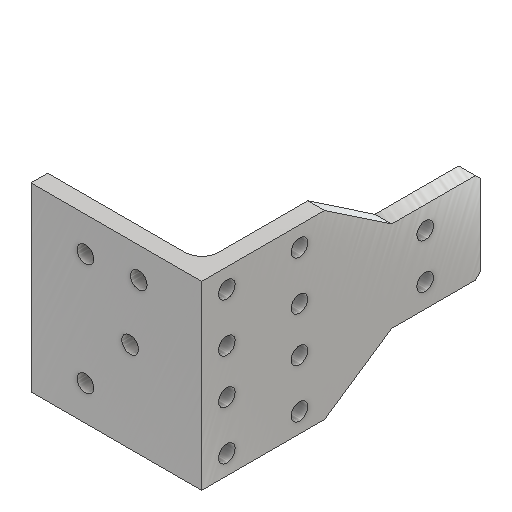
# Autodesk Inventor part: CNCM_X_Axiss_Carriage_Belt_and_Cable_Chain_Mount
Saved by Autodesk Inventor 2026.1 (Build 301233000, 233)
## iProperties
Created: 2016-03-27
Part Number: CNCM_X_Axiss_Carriage_Belt_and_Cable_Chain_Mount
Material: Ogólny
Document SubType Name: Modeling
Designer: Andrzej
Density: 1 g/cm^3
Appearance: Obrobione - aluminium
Mass: 6.52184 g
Surface Area: 50.6141 cm^2
Volume: 6.52184 cm^3
Author: Andrzej
Autodesk Inventor part; units mm, degrees
ref_plane "YZ Plane" through (0, 0, 0) normal (1, 0, 0) x (0, 1, 0)
ref_plane "XZ Plane" through (0, 0, 0) normal (0, 1, 0) x (-1, 0, 0)
ref_plane "XY Plane" through (0, 0, 0) normal (0, 0, 1) x (1, 0, 0)
sketch "Szkic1" plane through (0, 0, 0) normal (0, 0, 1) x (1, 0, 0)
  line L0 (-15.1556, -3.6171) -> (-15.1556, -6.6171)
  line L1 (-15.1556, -6.6171) -> (15.3944, -6.6171)
  line L2 (15.3944, -6.6171) -> (15.3944, 15.3829)
  line L3 (15.3944, 15.3829) -> (12.3944, 15.3829)
  line L4 (12.3944, 15.3829) -> (12.3944, -3.6171)
  line L5 (12.3944, -3.6171) -> (-15.1556, -3.6171)
  point P0 (0, 0)
  dimension "d0" = 3
  dimension "d1" = 30.55
  dimension "d2" = 22
  dimension "d3" = 3
  constraints: 12 end point, 5 perpendicular, 1 vertical
  measures "d0" distance of L0.start L0.end
  measures "d1" distance of L0.end L1.end
  measures "d2" distance of L1.end L2.end
  measures "d3" distance of L2.end L3.end
extrude "Wyciągnięcie proste1" add sketch "Szkic1" along normal blind 32.4
fillet "Zaokrąglenie1" radius 3 1 edges at (12.3944, -3.6171, 16.2)
sketch "Szkic3" plane through (15.3944, -6.6171, 32.4) normal (1, 0, 0) x (0, 0, -1)
  line L0 (32.4, 22) -> (0, 22) projected
  line L1 (0, 0) -> (0, 22) projected
  line L2 (32.4, 0) -> (0, 0) projected
  line L3 (32.4, 0) -> (32.4, 22) projected
  line L4 (32.4, 22) -> (0, 22) projected
  line L5 (24.3, 22) -> (8.1, 22)
  line L6 (8.1, 22) -> (8.1, 50)
  line L7 (8.1, 50) -> (24.3, 50)
  line L8 (24.3, 50) -> (24.3, 22)
  point P0 (32.4, 6.6171)
  dimension "d48" = 16.2
  dimension "d49" = 28
  dimension "d50" = 32.4
  dimension "d51" = 8.1
  constraints: 8 end point, 2 parallel, 1 horizontal, 1 perpendicular, 1 point on line
  measures "d48" distance of L6.end L7.end
  measures "d49" distance of L5.end L6.end
  measures "d50" distance between parallel lines of L1 L3
  measures "d51" distance between parallel lines of L3 L8
extrude "Wyciągnięcie proste3" add sketch "Szkic3" against normal blind 3 contours L0 L6 L7 L8
sketch "Szkic4" plane through (-15.1556, -6.6171, 0) normal (0, -1, 0) x (1, 0, 0)
  line L0 (0, 0) -> (30.55, 0) projected
  line L1 (30.55, 0) -> (30.55, 32.4) projected
  line L2 (0, 32.4) -> (30.55, 32.4) projected
  line L3 (0, 0) -> (0, 32.4) projected
  point P0 (15.1556, 0)
  point P1 (9.75, 26.2)
  point P2 (9.75, 6.2)
  point P3 (17.75, 16.2)
  dimension "d37" = 9.75
  dimension "d38" = 9.75
  dimension "d39" = 6.2
  dimension "d40" = 6.2
  dimension "d69" = 32.4
  dimension "d70" = 16.2
  dimension "d71" = 17.75
  measures "d37" distance from line of point (9.75, 26.2) L3
  measures "d38" distance from line of L3 point (9.75, 6.2)
  measures "d39" distance from line of L2 point (9.75, 26.2)
  measures "d40" distance from line of L0 point (9.75, 6.2)
  measures "d69" distance of L0.start L2.start
  measures "d70" distance from line of L2 point (17.75, 16.2)
  measures "d71" distance from line of L3 point (17.75, 16.2)
hole "Otwór2" at (-5.4056, -6.6171, 26.2) at (-5.4056, -6.6171, 6.2) at (2.5944, -6.6171, 16.2) direction (0, 1, 0) diameter 3 end through all
sketch "Szkic5" plane through (15.3944, -6.6171, 0) normal (1, 0, 0) x (0, 0, -1)
  line L0 (0, 0) -> (0, 22) projected
  line L1 (0, 22) -> (-8.1, 22) projected
  line L2 (-8.1, 22) -> (-8.1, 50) projected
  line L3 (-8.1, 50) -> (-24.3, 50) projected
  line L4 (-24.3, 50) -> (-24.3, 22) projected
  line L5 (-24.3, 22) -> (-32.4, 22) projected
  line L6 (-32.4, 0) -> (-32.4, 22) projected
  line L7 (0, 0) -> (-32.4, 0) projected
  point P0 (0, 6.6171)
  point P1 (-12.3, 40)
  point P2 (-20.3, 40)
  dimension "d52" = 10
  dimension "d53" = 10
  dimension "d54" = 4
  dimension "d55" = 4.2
  measures "d52" distance from line of L3 point (-12.3, 40)
  measures "d53" distance from line of L3 point (-20.3, 40)
  measures "d54" distance from line of L4 point (-20.3, 40)
  measures "d55" distance from line of L2 point (-12.3, 40)
hole "Otwór3" at (15.3944, 33.3829, 12.3) at (15.3944, 33.3829, 20.3) direction (-1, 0, 0) diameter 3 end through all
chamfer "Faza2" distance 1 angle 45 2 edges at (13.8944, 43.3829, 24.3) (13.8944, 43.3829, 8.1)
chamfer "Faza4" distance 8.1 distance2 12 1 edges at (13.8944, 15.3829, 24.3) measured on face at (14.3944, 15.3829, 27)
chamfer "Faza5" distance 8.1 distance2 12 1 edges at (13.8944, 15.3829, 8.1) measured on face at (14.3944, 15.3829, 2.7)
sketch "Szkic6" plane through (15.3944, -6.6171, 32.4) normal (1, 0, 0) x (0, 0, -1)
  circle A0 centre (20.1, 40) radius 1.5 projected
  circle A1 centre (12.1, 40) radius 1.5 projected
  line L0 (23.3, 50) -> (24.3, 49) projected
  line L1 (23.3, 50) -> (9.1, 50) projected
  line L2 (8.1, 49) -> (9.1, 50) projected
  line L3 (8.1, 49) -> (8.1, 34) projected
  line L4 (0, 22) -> (8.1, 34) projected
  line L5 (0, 0) -> (0, 22) projected
  line L6 (32.4, 0) -> (0, 0) projected
  line L7 (32.4, 0) -> (32.4, 22) projected
  line L8 (24.3, 34) -> (32.4, 22) projected
  line L9 (24.3, 34) -> (24.3, 49) projected
  point P0 (32.4, 6.6171)
  point P1 (3.5, 17.5)
  point P2 (3.5, 4.5)
  point P3 (28.9, 17.5)
  point P4 (28.9, 4.5)
  point P5 (35.2902, 42.5614)
  point P6 (12.2, 17.5)
  point P7 (12.2, 4.5)
  point P8 (20.2, 17.5)
  point P9 (20.2, 4.5)
  dimension "d79" = 3.5
  dimension "d80" = 3.5
  dimension "d81" = 3.5
  dimension "d82" = 3.5
  dimension "d83" = 4.5
  dimension "d84" = 4.5
  dimension "d85" = 13
  dimension "d86" = 13
  dimension "d87" = 8.7
  dimension "d88" = 8.7
  dimension "d89" = 8.7
  dimension "d90" = 8.7
  measures "d79" distance from line of L5 point (3.5, 17.5)
  measures "d80" distance from line of L5 point (3.5, 4.5)
  measures "d81" distance from line of L7 point (28.9, 4.5)
  measures "d82" distance from line of L7 point (28.9, 17.5)
  measures "d83" distance from line of L6 point (3.5, 4.5)
  measures "d84" distance from line of L6 point (28.9, 4.5)
  measures "d85" distance of point (3.5, 17.5) point (3.5, 4.5)
  measures "d86" distance of point (28.9, 17.5) point (28.9, 4.5)
  measures "d87" distance of point (3.5, 17.5) point (12.2, 17.5)
  measures "d88" distance of point (3.5, 4.5) point (12.2, 4.5)
  measures "d89" distance of point (28.9, 4.5) point (20.2, 4.5)
  measures "d90" distance of point (28.9, 17.5) point (20.2, 17.5)
hole "Otwór4" at (15.3944, 10.8829, 28.9) at (15.3944, -2.1171, 28.9) at (15.3944, 10.8829, 3.5) at (15.3944, -2.1171, 3.5) at (15.3944, 35.9442, -2.8902) at (15.3944, 10.8829, 20.2) at (15.3944, -2.1171, 20.2) at (15.3944, 10.8829, 12.2) at (15.3944, -2.1171, 12.2) direction (-1, 0, 0) diameter 3 end through all
sketch "Szkic7" plane through (-15.1556, -6.6171, 0) normal (0, -1, 0) x (1, 0, 0)
  circle A0 centre (9.75, 6.2) radius 1.5 projected
  circle A1 centre (9.75, 26.2) radius 1.5 projected
  circle A2 centre (17.75, 16.2) radius 1.5 projected
  line L0 (0, 0) -> (30.55, 0) projected
  line L1 (30.55, 0) -> (30.55, 32.4) projected
  line L2 (0, 32.4) -> (30.55, 32.4) projected
  line L3 (0, 0) -> (0, 32.4) projected
  point P0 (15.1556, 0)
  point P1 (19.3, 26.96)
  dimension "d98" = 5.44
  dimension "d99" = 19.3
  measures "d98" distance from line of L2 point (19.3, 26.96)
  measures "d99" distance from line of L3 point (19.3, 26.96)
hole "Otwór5" at (4.1444, -6.6171, 26.96) direction (0, 1, 0) diameter 3 depth 8 tip angle 118
equation "\"d51\" = -0.5 * d48 + 0.5 * d50"
equation "\"d38\" = d37"
equation "\"d40\" = d39"
equation "\"d70\" = 0.5 * d69"
equation "\"d53\" = d52"
equation "\"d80\" = d79"
equation "\"d81\" = d79"
equation "\"d82\" = d79"
equation "\"d84\" = d83"
equation "\"d86\" = d85"
equation "\"d88\" = d87"
equation "\"d89\" = d87"
equation "\"d90\" = d87"
